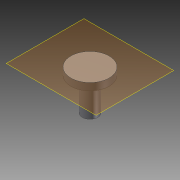
# Autodesk Inventor part: ArmPivot
Saved by Autodesk Inventor 2012 (Build 160160000, 160)
## iProperties
Created: 2011-10-28
Part Number: ArmPivot
Material: Default
Document SubType Name: Modeling
Designer: KuttaA
Density: 1 g/cm^3
Author: KuttaA
Autodesk Inventor part; units mm, degrees
ref_plane "YZ Plane" through (0, 0, 0) normal (1, 0, 0) x (0, 1, 0)
ref_plane "XZ Plane" through (0, 0, 0) normal (0, 1, 0) x (-1, 0, 0)
ref_plane "XY Plane" through (0, 0, 0) normal (0, 0, 1) x (1, 0, 0)
ref_plane "Work Plane1" through (12.5, -13.8, 2.5) normal (0, 0, 1) x (1, 0, 0)
sketch "Sketch2" plane through (12.5, -13.8, 2.5) normal (0, 0, 1) x (1, 0, 0)
  circle A0 centre (-12.5, 13.8) radius 6.15 projected
  circle A1 centre (-12.5, 13.8) radius 5.85
  dimension "d0" = 0.3
  constraints: 1 centre point, 1 coincident
  measures "d0" radial gap between concentric circles of A0 A1
extrude "Extrusion1" add sketch "Sketch2" against normal blind 2.2 contours A1
sketch "Sketch3" plane through (0, 0, 0.3) normal (0, 0, -1) x (-1, 0, 0)
  circle A0 centre (0, 0) radius 5.85 projected
  circle A1 centre (0, 0) radius 2.65 projected
  circle A2 centre (0, 0) radius 2.35
  dimension "d3" = 0.3
  constraints: 1 centre point, 1 coincident
  measures "d3" radial gap between concentric circles of A1 A2
extrude "Extrusion2" add sketch "Sketch3" along normal blind 10 contours A2
body "Solid1"
